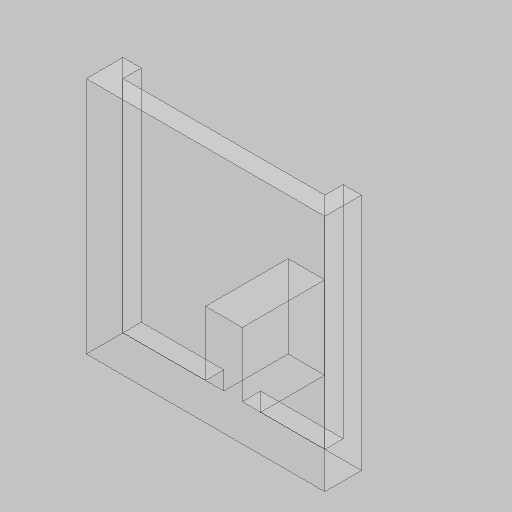
# Autodesk Inventor part: NV_module_lid_2
Saved by Autodesk Inventor 2026.1 (Build 301233020, 233B)
## iProperties
Created: 2026-01-23
Part Number: NV_module_lid_2
Material: PET Plastic
Document SubType Name: Modeling
Designer: samuel
Density: 1.541 g/cm^3
Appearance: Polycarbonate - Clear
Author: samuel
Autodesk Inventor part; units mm, degrees
ref_plane "YZ Plane" through (0, 0, 0) normal (1, 0, 0) x (0, 1, 0)
ref_plane "XZ Plane" through (0, 0, 0) normal (0, 1, 0) x (-1, 0, 0)
ref_plane "XY Plane" through (0, 0, 0) normal (0, 0, 1) x (1, 0, 0)
sketch "Sketch1" plane through (0, 0, 0) normal (0, 0, 1) x (1, 0, 0)
  line L0 (-6.5, -6.5) -> (6.5, -6.5)
  line L1 (6.5, -6.5) -> (6.5, 6.5)
  line L2 (6.5, 6.5) -> (-6.5, 6.5)
  line L3 (-6.5, 6.5) -> (-6.5, -6.5)
  line L4 (-6.5, -6.5) -> (6.5, 6.5) construction
  line L5 (6.5, -6.5) -> (-6.5, 6.5) construction
  line L6 (-5.5, 5.5) -> (5.5, 5.5)
  line L7 (5.5, 5.5) -> (5.5, -5.5)
  line L8 (5.5, -5.5) -> (-5.5, -5.5)
  line L9 (-5.5, -5.5) -> (-5.5, 5.5)
  point P0 (0, 0)
  dimension "d0" = 13
  dimension "d1" = 13
  dimension "d2" = 1
  constraints: 20 end point, 4 parallel, 2 midpoint, 2 perpendicular, 1 horizontal, 3 other
  measures "d0" distance of L2.end L1.end
  measures "d1" distance of L1.end L0.end
  measures "d2" distance between parallel lines of L2 L6
extrude "Extrusion1" add sketch "Sketch1" along normal blind 2 contours L3 L2 L1 L0 | L6 L7 L8 L9
extrude "Extrusion2" cut sketch "Sketch1" along normal blind 1 contours L6 L7 L8 L9
sketch "Sketch2" plane through (0, 0, 2) normal (0, 0, 1) x (1, 0, 0)
  line L0 (-6.5, -6.5) -> (6.5, -6.5) projected
  line L1 (-1, -6.5) -> (1, -6.5)
  line L2 (1, -6.5) -> (1, -2)
  line L3 (1, -2) -> (-1, -2)
  line L4 (-1, -2) -> (-1, -6.5)
  point P0 (0, 0)
  point P1 (0, -6.5)
  dimension "d7" = 2
  dimension "d8" = 4.5
  dimension "d9" = 1
  constraints: 8 end point, 2 parallel, 1 horizontal, 1 midpoint, 1 perpendicular, 1 point on line
  measures "d7" distance of L3.end L2.end
  measures "d8" distance of L2.end L1.end
  measures "d9" distance from line of point (0, -6.5) L4
extrude "Extrusion3" add sketch "Sketch2" against normal blind 5.5
sketch "Sketch3" plane through (0, 0, 0) normal (0, 0, -1) x (-1, 0, 0)
  line L0 (-5.5, 5.5) -> (5.5, 5.5) projected
  line L1 (-6.5, 6.5) -> (6.5, 6.5) projected
  line L2 (-5.5, 5.5) -> (5.5, 5.5)
  line L3 (5.5, 5.5) -> (5.5, 6.5)
  line L4 (5.5, 6.5) -> (-5.5, 6.5)
  line L5 (-5.5, 6.5) -> (-5.5, 5.5)
  point P0 (0, 0)
  dimension "d12" = 11
  constraints: 8 end point, 2 parallel, 1 horizontal, 1 perpendicular, 1 point on line
  measures "d12" distance of L4.end L3.end
extrude "Extrusion4" cut sketch "Sketch3" against normal blind 1
body "Solid1"
